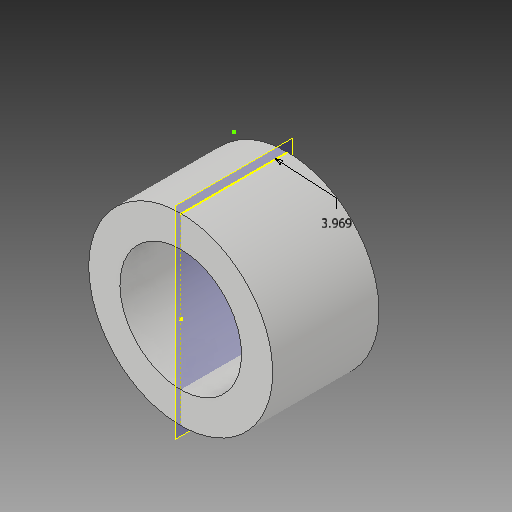
# Autodesk Inventor part: Bearing 608 Inner Race
Saved by Autodesk Inventor 2018 (Build 220112000, 112)
## iProperties
Created: 2017-09-15
Part Number: Bearing 608 Inner Race
Material: Generic
Document SubType Name: Modeling
Designer: Rus
Density: 1 g/cm^3
Appearance: Default
Author: Rus
Autodesk Inventor part; units mm, degrees
ref_plane "YZ Plane" through (0, 0, 0) normal (1, 0, 0) x (0, 1, 0)
ref_plane "XZ Plane" through (0, 0, 0) normal (0, 1, 0) x (-1, 0, 0)
ref_plane "XY Plane" through (0, 0, 0) normal (0, 0, 1) x (1, 0, 0)
sketch "Sketch1" plane through (0, 0, 0) normal (0, 0, 1) x (1, 0, 0)
  circle A0 centre (0, 0) radius 4
  circle A1 centre (0, 0) radius 6.05
  line L0 (0, -4) -> (0, -6.05)
  line L1 (4, 0) -> (6.05, 0) construction
  line L2 (0, 4) -> (0, 6.05)
  dimension "d0" = 8
  dimension "d1" = 12.1
  dimension "d2" = 90
  dimension "d3" = 90
  dimension "d4" = 4
  dimension "d5" = 4
  constraints: 6 end point, 6 point on circle, 2 centre point, 2 coincident, 1 horizontal, 1 vertical
  measures "d0" diameter of A0
  measures "d1" diameter of A1
  measures "d2" angle of L1 L2
  measures "d3" angle of L0 L1
  measures "d4" distance from line of L1.start L0
  measures "d5" horizontal distance of L1.start L2.start
sketch "Sketch1 outline for Extrusion1" plane through (0, 0, 0) normal (0, 0, 1) x (1, 0, 0)
  line L0 (0, -6.05) -> (0, -4)
  arc A0 (0, 6.05) -> (0, -6.05) centre (0, 0) ccw
  line L1 (0, 4) -> (0, 6.05)
  arc A1 (0, -4) -> (0, 4) centre (0, 0) cw
extrude "Extrusion1" add sketch "Sketch1 outline for Extrusion1" against normal blind 7
ref_plane "Work Plane1" through (0, 4, 0) normal (-1, 0, 0) x (0, 1, 0)
mirror "Mirror1" about plane through (0, 6.05, 0) normal (1, 0, 0) of "Extrusion1"
sketch "Sketch3" plane through (0, 4, 0) normal (-1, 0, 0) x (0, 1, 0)
  line L0 (2.05, 0) -> (2.05, 7)
  arc A0 (2.05, 6.230644) -> (2.05, 0.769356) centre (4.930028, 3.5) ccw
  line L1 (0.961278, 3.5) -> (0.961278, 0) construction
  line L2 (-10.05, 0) -> (2.05, 0) construction
  line L3 (0.961278, 3.5) -> (0.961278, 7) construction
  line L4 (-10.05, 7) -> (2.05, 7) construction
  line L5 (2.05, 0.769356) -> (2.05, 6.230644) construction
  point P0 (-4, 0)
  dimension "d8" = 3.96875
  constraints: 6 end point, 5 point on line, 3 point on circle, 2 collinear, 1 centre point, 1 vertical
  measures "d8" radius of A0
body "Solid1"
